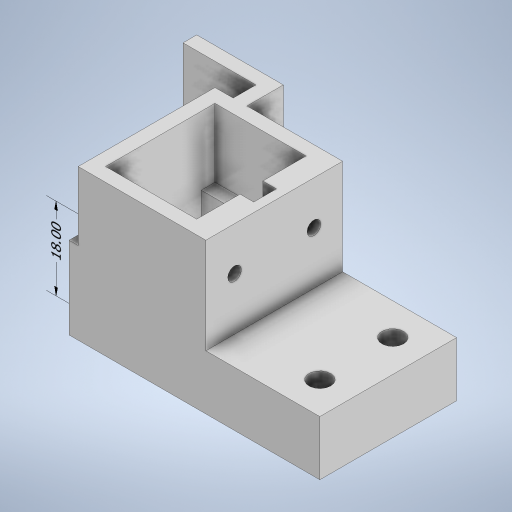
# Autodesk Inventor part: Soporte_motor
Saved by Autodesk Inventor 2023 (Build 270158000, 158)
## iProperties
Created: 2023-06-06
Part Number: Soporte_motor
Material: Genérico
Document SubType Name: Modeling
Designer: sergi
Density: 1 g/cm^3
Appearance: Valor por defecto
Author: sergi
Autodesk Inventor part; units mm, degrees
ref_plane "YZ Plane" through (0, 0, 0) normal (1, 0, 0) x (0, 1, 0)
ref_plane "XZ Plane" through (0, 0, 0) normal (0, 1, 0) x (-1, 0, 0)
ref_plane "XY Plane" through (0, 0, 0) normal (0, 0, 1) x (1, 0, 0)
sketch "Boceto1" plane through (0, 0, 0) normal (0, 1, 0) x (-1, 0, 0)
  line L0 (-10, -9) -> (10, -9)
  line L1 (10, -9) -> (10, 9)
  line L2 (10, 9) -> (-10, 9)
  line L3 (-10, 9) -> (-10, -9)
  line L4 (-10, -9) -> (10, 9) construction
  line L5 (10, -9) -> (-10, 9) construction
  line L6 (-15, -15) -> (15, -15)
  line L7 (15, -15) -> (15, 15)
  line L8 (15, 15) -> (-15, 15)
  line L9 (-15, 15) -> (-15, -15)
  line L10 (-15, -15) -> (15, 15) construction
  line L11 (15, -15) -> (-15, 15) construction
  point P0 (0, 0)
  dimension "d0" = 20
  dimension "d1" = 18
  dimension "d2" = 30
  dimension "d3" = 30
  constraints: 24 end point, 4 midpoint, 4 parallel, 2 horizontal, 2 perpendicular
  measures "d0" distance of L2.end L1.end
  measures "d1" distance of L0.end L1.end
  measures "d2" distance of L8.end L7.end
  measures "d3" distance of L6.end L7.end
extrude "Extrusión1" add sketch "Boceto1" along normal blind 18
sketch "Boceto2" plane through (0, 18, 0) normal (0, 1, 0) x (1, 0, 0)
  line L0 (10, 12) -> (-10, 12)
  line L1 (-10, 12) -> (-10, -12)
  line L2 (-10, -12) -> (10, -12)
  line L3 (10, -12) -> (10, 12)
  line L4 (10, 12) -> (-10, -12) construction
  line L5 (-10, 12) -> (10, -12) construction
  line L6 (-15, 15) -> (-15, -15) projected
  line L7 (-15, -15) -> (15, -15) projected
  line L8 (15, -15) -> (15, 15) projected
  line L9 (15, 15) -> (-15, 15) projected
  line L10 (10, 9) -> (10, -9) projected
  line L11 (10, -9) -> (-10, -9) projected
  line L12 (-10, -9) -> (-10, 9) projected
  line L13 (-10, 9) -> (10, 9) projected
  point P0 (0, 0)
  dimension "d6" = 20
  dimension "d7" = 24
  constraints: 12 end point, 2 midpoint, 2 parallel, 1 horizontal, 1 perpendicular
  measures "d6" distance of L2.end L1.end
  measures "d7" distance of L0.end L1.end
extrude "Extrusión2" add sketch "Boceto2" along normal blind 15
sketch "Boceto4" plane through (15, 0, 15) normal (1, 0, 0) x (0, 0, -1)
  line L0 (30, 0) -> (30, 33) projected
  line L1 (0, 0) -> (0, 33) projected
  line L2 (30, 0) -> (0, 0)
  line L3 (0, 0) -> (0, 12)
  line L4 (0, 12) -> (30, 12)
  line L5 (30, 12) -> (30, 0)
  point P0 (15, 0)
  dimension "d13" = 12
  constraints: 8 end point, 2 parallel, 1 horizontal, 1 perpendicular, 1 point on line
  measures "d13" distance between parallel lines of L2 L4
extrude "Extrusión4" add sketch "Boceto4" along normal blind 25
sketch "Boceto5" plane through (15, 12, 15) normal (0, 1, 0) x (1, 0, 0)
  circle A0 centre (18, 7) radius 2.3813
  circle A1 centre (18, 23) radius 2.3812
  line L0 (25, 30) -> (25, 0) projected
  line L1 (0, 0) -> (25, 0) projected
  line L2 (0, 30) -> (25, 30) projected
  point P0 (-15, 15)
  dimension "d16" = 4.7625
  dimension "d17" = 4.7625
  dimension "d18" = 7
  dimension "d19" = 7
  dimension "d20" = 7
  dimension "d21" = 7
  constraints: 2 centre point
  measures "d16" diameter of A0
  measures "d17" diameter of A1
  measures "d18" distance from line of L0 A0.centre
  measures "d19" distance from line of L1 A0.centre
  measures "d20" distance from line of L2 A1.centre
  measures "d21" distance from line of L0 A1.centre
extrude "Extrusión5" cut sketch "Boceto5" against normal through all
sketch "Boceto6" plane through (0, 33, 0) normal (0, 1, 0) x (1, 0, 0)
  line L0 (10, 9) -> (10, -9) projected
  line L1 (10, -2.5) -> (13, -2.5)
  line L2 (13, -2.5) -> (13, 2.5)
  line L3 (13, 2.5) -> (10, 2.5)
  line L4 (10, 2.5) -> (10, -2.5)
  point P0 (0, 0)
  point P1 (10, 0)
  dimension "d24" = 5
  dimension "d25" = 3
  constraints: 8 end point, 2 parallel, 1 horizontal, 1 horizontal alignment, 1 midpoint, 1 perpendicular, 1 point on line
  measures "d24" distance between parallel lines of L3 L1
  measures "d25" distance of L2.end L3.end
extrude "Extrusión6" cut sketch "Boceto6" against normal blind 5
sketch "Boceto7" plane through (15, 33, 15) normal (1, 0, 0) x (0, 0, -1)
  circle A0 centre (6.3, -9.5) radius 1.5
  circle A1 centre (23.7, -9.5) radius 1.5
  line L0 (30, -21) -> (0, -21) projected
  line L1 (0, -21) -> (0, 0) projected
  line L2 (30, -21) -> (30, 0) projected
  line L3 (6.3, -9.5) -> (23.7, -9.5)
  line L4 (0, -33) -> (30, -33) projected
  point P0 (15, -33)
  point P1 (15, -9.5)
  point P2 (15, -33)
  dimension "d28" = 3
  dimension "d29" = 3
  dimension "d30" = 11.5
  dimension "d32" = 11.5
  dimension "d34" = 17.4
  constraints: 2 centre point, 2 end point, 2 midpoint, 1 vertical alignment
  measures "d28" diameter of A0
  measures "d29" diameter of A1
  measures "d30" distance from line of L0 L3.start
  measures "d32" distance from line of L0 L3.end
  measures "d34" distance of L3.start L3.end
extrude "Extrusión7" cut sketch "Boceto7" against normal blind 5
sketch "Boceto8" plane through (-15, 0, -15) normal (-1, 0, 0) x (0, 0, 1)
  line L0 (0, 33) -> (30, 33) projected
  line L1 (30, 12) -> (30, 33) projected
  line L2 (0, 33) -> (30, 33)
  line L3 (30, 33) -> (30, 18)
  line L4 (30, 18) -> (0, 18)
  line L5 (0, 18) -> (0, 33)
  point P0 (15, 0)
  dimension "d43" = 15
  constraints: 8 end point, 2 parallel, 1 horizontal, 1 perpendicular, 1 point on line
  measures "d43" distance between parallel lines of L4 L0
extrude "Extrusión8" cut sketch "Boceto8" against normal blind 2
sketch "Boceto9" plane through (40, 0, -15) normal (0, 0, -1) x (-1, 0, 0)
  line L0 (50, 33) -> (30, 33) projected
  line L1 (46, 33) -> (49, 33)
  line L2 (49, 33) -> (49, 0)
  line L3 (49, 0) -> (46, 0)
  line L4 (46, 0) -> (46, 33)
  line L5 (53, 18) -> (53, 33) projected
  point P0 (40, 0)
  dimension "d46" = 3
  dimension "d47" = 4
  constraints: 8 end point, 2 parallel, 1 horizontal, 1 perpendicular, 1 point on line
  measures "d46" distance between parallel lines of L2 L4
  measures "d47" distance between parallel lines of L5 L2
extrude "Extrusión9" add sketch "Boceto9" along normal blind 8
sketch "Boceto10" plane through (-9, 0, -15) normal (-1, 0, 0) x (0, 0, 1)
  line L0 (0, 33) -> (-8, 33) projected
  line L1 (0, 0) -> (-8, 0) projected
  line L2 (-8, 33) -> (-5, 33)
  line L3 (-5, 33) -> (-5, 0)
  line L4 (-5, 0) -> (-8, 0)
  line L5 (-8, 0) -> (-8, 33)
  point P0 (15, 0)
  point P1 (-8, 0)
  dimension "d50" = 3
  constraints: 8 end point, 2 parallel, 1 horizontal, 1 perpendicular, 1 point on line
  measures "d50" distance between parallel lines of L3 L5
extrude "Extrusión10" add sketch "Boceto10" along normal blind 16
sketch "Boceto11" plane through (40, 0, -23) normal (0, 0, -1) x (-1, 0, 0)
  circle A0 centre (57, 22) radius 1.5
  line L0 (46, 33) -> (65, 33) projected
  line L1 (46, 33) -> (46, 0) projected
  point P0 (40, 0)
  dimension "d53" = 3
  dimension "d54" = 11
  dimension "d55" = 11
  constraints: 1 centre point
  measures "d53" diameter of A0
  measures "d54" distance from line of L0 A0.centre
  measures "d55" distance from line of L1 A0.centre
extrude "Extrusión11" cut sketch "Boceto11" against normal up to surface (3 mm away)
